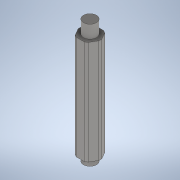
# Autodesk Inventor part: DriveShaft
Saved by Autodesk Inventor 2020 (Build 240168000, 168)
## iProperties
Created: 2019-05-28
Part Number: DriveShaft
Material: Steel, Alloy
Document SubType Name: Modeling
Designer: Connor
Density: 7.73 g/cm^3
Appearance: Semi-Polished
Author: Connor
Autodesk Inventor part; units mm, degrees
ref_plane "YZ Plane" through (0, 0, 0) normal (1, 0, 0) x (0, 1, 0)
ref_plane "XZ Plane" through (0, 0, 0) normal (0, 1, 0) x (-1, 0, 0)
ref_plane "XY Plane" through (0, 0, 0) normal (0, 0, 1) x (1, 0, 0)
sketch "Sketch1" plane through (0, 0, 0) normal (0, 1, 0) x (-1, 0, 0)
  line L0 (-5.4993, 0) -> (-2.7496, 4.7625)
  line L1 (-2.7496, 4.7625) -> (2.7496, 4.7625)
  line L2 (2.7496, 4.7625) -> (5.4993, 0)
  line L3 (5.4993, 0) -> (2.7496, -4.7625)
  line L4 (2.7496, -4.7625) -> (-2.7496, -4.7625)
  line L5 (-2.7496, -4.7625) -> (-5.4993, 0)
  circle A0 centre (0, 0) radius 5.125
  point P0 (1.8932, -4.7625)
  point P1 (3.1778, -4.0208)
  point P2 (5.071, -0.7417)
  point P3 (5.071, 0.7417)
  point P4 (3.1778, 4.0208)
  point P5 (1.8932, 4.7625)
  point P6 (-1.8932, 4.7625)
  point P7 (-3.1778, 4.0208)
  point P8 (-5.071, 0.7417)
  point P9 (-5.071, -0.7417)
  point P10 (-3.1778, -4.0208)
  point P11 (-1.8932, -4.7625)
  dimension "d0" = 9.525
  dimension "d1" = 10.25
  constraints: 12 end point, 2 coincident, 1 centre point, 13 other
  measures "d0" distance between parallel lines of L1 L4
  measures "d1" diameter of A0
extrude "Extrusion1" add sketch "Sketch1" along normal blind 60.325 contours L0 A0 L1 L2 L3 L4 L5
sketch "Sketch2" plane through (0, 0, 0) normal (0, -1, 0) x (1, 0, 0)
  circle A0 centre (0, 0) radius 3.175
  arc A1 (3.1778, 4.0208) -> (1.8932, 4.7625) centre (0, 0) ccw projected
  line L0 (-1.8932, 4.7625) -> (1.8932, 4.7625) projected
  arc A2 (-1.8932, 4.7625) -> (-3.1778, 4.0208) centre (0, 0) ccw projected
  line L1 (-5.071, 0.7417) -> (-3.1778, 4.0208) projected
  arc A3 (-5.071, 0.7417) -> (-5.071, -0.7417) centre (0, 0) ccw projected
  line L2 (-3.1778, -4.0208) -> (-5.071, -0.7417) projected
  arc A4 (-3.1778, -4.0208) -> (-1.8932, -4.7625) centre (0, 0) ccw projected
  line L3 (1.8932, -4.7625) -> (-1.8932, -4.7625) projected
  arc A5 (1.8932, -4.7625) -> (3.1778, -4.0208) centre (0, 0) ccw projected
  line L4 (5.071, -0.7417) -> (3.1778, -4.0208) projected
  arc A6 (5.071, -0.7417) -> (5.071, 0.7417) centre (0, 0) ccw projected
  line L5 (3.1778, 4.0208) -> (5.071, 0.7417) projected
  dimension "d4" = 6.35
  constraints: 1 centre point, 1 coincident
  measures "d4" diameter of A0
extrude "Extrusion2" cut sketch "Sketch2" against normal blind 3.175
sketch "Sketch3" plane through (0, 60.325, 0) normal (0, 1, 0) x (1, 0, 0)
  line L0 (5.071, 0.7417) -> (3.1778, 4.0208) projected
  arc A0 (3.1778, 4.0208) -> (1.8932, 4.7625) centre (0, 0) ccw projected
  line L1 (1.8932, 4.7625) -> (-1.8932, 4.7625) projected
  arc A1 (-1.8932, 4.7625) -> (-3.1778, 4.0208) centre (0, 0) ccw projected
  line L2 (-3.1778, 4.0208) -> (-5.071, 0.7417) projected
  arc A2 (-5.071, 0.7417) -> (-5.071, -0.7417) centre (0, 0) ccw projected
  line L3 (-5.071, -0.7417) -> (-3.1778, -4.0208) projected
  arc A3 (-3.1778, -4.0208) -> (-1.8932, -4.7625) centre (0, 0) ccw projected
  line L4 (-1.8932, -4.7625) -> (1.8932, -4.7625) projected
  arc A4 (1.8932, -4.7625) -> (3.1778, -4.0208) centre (0, 0) ccw projected
  line L5 (3.1778, -4.0208) -> (5.071, -0.7417) projected
  arc A5 (5.071, -0.7417) -> (5.071, 0.7417) centre (0, 0) ccw projected
  circle A6 centre (0, 0) radius 3.175
  dimension "d7" = 6.35
  constraints: 1 centre point, 1 coincident
  measures "d7" diameter of A6
extrude "Extrusion3" cut sketch "Sketch3" against normal blind 6.35
body "Solid1"
